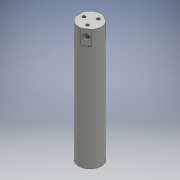
# Autodesk Inventor part: shaft2
Saved by Autodesk Inventor 2016 SP1 (Build 200210100, 210)
## iProperties
Created: 2017-01-24
Part Number: shaft2
Material: 一般
Document SubType Name: Modeling
Designer: p_admin
Density: 1 g/cm^3
Appearance: 既定
Author: p_admin
Autodesk Inventor part; units mm, degrees
ref_plane "YZ Plane" through (0, 0, 0) normal (1, 0, 0) x (0, 1, 0)
ref_plane "XZ Plane" through (0, 0, 0) normal (0, 1, 0) x (-1, 0, 0)
ref_plane "XY Plane" through (0, 0, 0) normal (0, 0, 1) x (1, 0, 0)
sketch "スケッチ1" plane through (0, 0, 0) normal (0, 0, 1) x (1, 0, 0)
  circle A0 centre (0, 0) radius 7.5
  dimension "d0" = 15
  constraints: 1 centre point, 1 coincident
  measures "d0" diameter of A0
extrude "押し出し1" add sketch "スケッチ1" along normal blind 30
sketch "スケッチ2" plane through (0, 0, 30) normal (0, 0, 1) x (1, 0, 0)
  circle A0 centre (0, 0) radius 7.5 projected
  arc A1 (-7.0477, 2.5652) -> (-7.0477, -2.5652) centre (0, 0) ccw
  line L0 (0, 0) -> (-7.0477, 2.5652) construction
  line L1 (0, 0) -> (7.5, 0) construction
  line L2 (0, 0) -> (-7.0477, -2.5652) construction
  line L3 (-7.0477, 2.5652) -> (-7.0477, -2.5652)
  line L4 (-7.5, 0) -> (4.8374, 7.123)
  line L5 (-7.5, 0) -> (6.746, 0) construction
  line L6 (-7.5, 0) -> (4.8374, -7.123)
  line L7 (-7.5, 0) -> (6.746, 0) construction
  arc A2 (5.7453, 4.8209) -> (1.3024, 7.3861) centre (0, 0) ccw
  line L8 (0, 0) -> (1.3024, 7.3861) construction
  line L9 (0, 0) -> (7.5, 0) construction
  line L10 (0, 0) -> (5.7453, 4.8209) construction
  arc A3 (1.3024, -7.3861) -> (5.7453, -4.8209) centre (0, 0) ccw
  line L11 (0, 0) -> (5.7453, -4.8209) construction
  line L12 (0, 0) -> (7.5, 0) construction
  line L13 (0, 0) -> (1.3024, -7.3861) construction
  circle A4 centre (0, 0) radius 7.5
  line L14 (1.3024, 7.3861) -> (5.7453, 4.8209)
  line L15 (5.7453, -4.8209) -> (1.3024, -7.3861)
  dimension "d15" = 160
  dimension "d16" = 40
  dimension "d17" = 30
  dimension "d18" = 30
  dimension "d19" = 80
  dimension "d20" = 40
  dimension "d21" = 40
  dimension "d22" = 40
  constraints: 32 end point, 9 point on circle, 5 equal length, 5 horizontal, 4 centre point, 4 coincident, 3 other
  measures "d15" angle of L1 L0
  measures "d16" angle of L0 L2
  measures "d17" angle of L5 L4
  measures "d18" angle of L6 L7
  measures "d19" angle of L9 L8
  measures "d20" angle of L10 L8
  measures "d21" angle of L11 L12
  measures "d22" angle of L13 L11
extrude "押し出し2" add sketch "スケッチ2" along normal blind 10 contours A0 L15 L6 L3 L4 L14 | L4 L3 A0 L14 | L15 A0 L3 L6
sketch "スケッチ3" plane through (5.7453, -4.8209, 30) normal (0.5, -0.8660254, 0) x (0.8660254, 0.5, 0)
  circle A0 centre (-2.5652, 5) radius 2
  line L0 (-5.1303, 10) -> (0, 10) projected
  point P0 (-2.5652, -30)
  dimension "d25" = 4
  dimension "d26" = 5
  constraints: 1 centre point
  measures "d25" diameter of A0
  measures "d26" distance from line of L0 A0.centre
sketch "スケッチ4" plane through (-7.0477, -2.5652, 30) normal (-1, 0, 0) x (0, 0, 1)
  circle A0 centre (5, 2.5652) radius 2
  line L0 (10, 5.1303) -> (10, 0) projected
  point P0 (-30, 2.5652)
  dimension "d27" = 4
  dimension "d28" = 5
  constraints: 1 centre point
  measures "d27" diameter of A0
  measures "d28" distance from line of L0 A0.centre
sketch "スケッチ5" plane through (1.3024, 7.3861, 40) normal (0.5, 0.8660254, 0) x (0.8660254, -0.5, 0)
  circle A0 centre (2.5652, 5) radius 2
  line L0 (5.1303, 0) -> (0, 0) projected
  point P0 (2.5652, 40)
  dimension "d29" = 4
  dimension "d30" = 5
  constraints: 1 centre point
  measures "d29" diameter of A0
  measures "d30" distance from line of L0 A0.centre
extrude "押し出し3" cut sketch "スケッチ5" against normal blind 6
extrude "押し出し4" cut sketch "スケッチ3" against normal blind 6
extrude "押し出し5" cut sketch "スケッチ4" against normal blind 6
thread "ねじ1" size "M4x0.7" class "6H" standard "ISO Metric profile" full length
thread "ねじ2" size "M4x0.7" class "6H" standard "ANSI Metric M Profile" full length
thread "ねじ3" size "M4x0.7" class "6H" standard "ANSI Metric M Profile" full length
sketch "スケッチ6" plane through (0, 0, 0) normal (0, 0, -1) x (-1, 0, 0)
  line L0 (-2.5, 5.15) -> (2.5, 5.15)
  line L1 (-2.5, 5.15) -> (2.5, 5.15) construction
  line L2 (-2.5, 5.15) -> (-2.5, 7.45)
  line L3 (-2.5, 5.15) -> (-0.2, 5.15) construction
  arc A0 (-1.3024, 7.3861) -> (-5.7453, 4.8209) centre (0, 0) ccw projected
  line L4 (-2.5, 7.0711) -> (-2.5, 4.7711)
  line L5 (-2.5, 4.7711) -> (2.5, 4.7711)
  line L6 (2.5, 4.7711) -> (2.5, 7.0711)
  circle A1 centre (0, 0) radius 7.5 projected
  arc A2 (-2.5, 7.0711) -> (2.5, 7.0711) centre (0, 0) ccw
  dimension "d43" = 5
  dimension "d44" = 0
  dimension "d45" = 2.5
  dimension "d46" = 2.3
  dimension "d47" = 90
  dimension "d48" = 2.3
  dimension "d49" = 5
  dimension "d50" = 90
  constraints: 14 end point, 4 point on circle, 3 horizontal, 2 equal length, 2 point on line, 1 centre point, 1 coincident, 1 concentric, 1 parallel, 1 vertical
  measures "d43" distance of L0.start L0.end
  measures "d44" distance between parallel lines of L0 L1
  measures "d45" horizontal distance of L1.end point (0, 0)
  measures "d46" distance of L0.start L2.end
  measures "d47" angle of L3 L2
  measures "d48" distance of L4.start L4.end
  measures "d49" distance of L4.end L5.end
  measures "d50" angle of L6 L5
extrude "押し出し6" add sketch "スケッチ6" along normal blind 40 contours L4 L5 L6 A1 A0 L2
sketch "スケッチ7" plane through (0, 0, 40) normal (0, 0, 1) x (1, 0, 0)
  circle A0 centre (-4.0477, -0.016) radius 1
  line L0 (-7.0477, 2.5652) -> (-7.0477, -2.5652) projected
  circle A1 centre (0, 0) radius 4.0477
  circle A2 centre (1.9372, -3.554) radius 1
  circle A3 centre (2.01, 3.5134) radius 1
  line L1 (-4.0477, -0.016) -> (2.01, -3.5134)
  line L2 (-4.0477, -0.016) -> (2.9472, -0.016) construction
  line L3 (2.01, -3.5134) -> (2.01, 3.5134)
  dimension "d53" = 2
  dimension "d54" = 3
  dimension "d55" = 2
  dimension "d56" = 2
  dimension "d57" = 30
  constraints: 6 end point, 4 centre point, 4 point on circle, 1 coincident, 1 equal length, 1 horizontal, 1 vertical
  measures "d53" diameter of A0
  measures "d54" distance from line of L1.start L0
  measures "d55" diameter of A2
  measures "d56" diameter of A3
  measures "d57" angle of L1 L2
hole "穴1" at (-4.0477, -0.016, 40) at (2.01, 3.5134, 40) at (1.9372, -3.554, 40) direction (0, 0, -1) diameter 2 depth 10 tip angle 118
thread "ねじ4" size "M2x0.4" class "6H" standard "ANSI Metric M Profile" full length
thread "ねじ5" size "M2x0.4" class "6H" standard "ANSI Metric M Profile" full length
thread "ねじ6" size "M2x0.4" class "6H" standard "ANSI Metric M Profile" full length
thread "ねじ7" size "M2x0.4" class "6H" standard "ANSI Metric M Profile" full length
thread "ねじ8" size "M2x0.4" class "6H" standard "ANSI Metric M Profile" full length
thread "ねじ9" size "M2x0.4" class "6H" standard "ANSI Metric M Profile" full length
